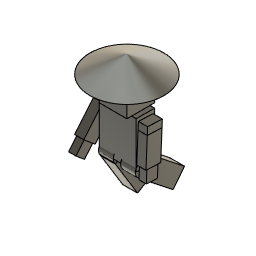
Body v3 (Autodesk Fusion 360 design; units mm, degrees)
Autodesk Fusion 360 part; units mm, degrees
sketch "Skizze2" plane through (0, 0, 0) normal (0, 0, 1) x (1, 0, 0)
  line L0 (-10, 5) -> (10, 5)
  line L1 (10, 5) -> (10, -5)
  line L2 (10, -5) -> (-10, -5)
  line L3 (-10, -5) -> (-10, 5)
  line L4 (-10, 0) -> (10, 0) construction
  line L5 (0, 5) -> (0, -5) construction
  dimension "d1" = 20
  dimension "d2" = 10
  constraint horizontal L0
  constraint vertical L1
  constraint horizontal L2
  constraint vertical L3
  constraint midpoint L3 L4.start
  constraint midpoint L1 L4.end
  constraint midpoint L0 L5.start
  constraint midpoint L2 L5.end
  constraint coincident origin L5
  constraint coincident origin L4
  measures "d1" distance of L0.start L0.end
  measures "d2" distance of L0 L2
extrude "Extrusion1" add sketch "Skizze2" along normal blind 25 makes body 1 in component "Body"
sketch "Skizze3" plane through (0, 0, 25) normal (0, 0, 1) x (-1, 0, 0)
  line L0 (10, 5) -> (-10, 5)
  line L1 (-10, 5) -> (-10, -5)
  line L2 (-10, -5) -> (10, -5)
  line L3 (10, -5) -> (10, 5)
  line L4 (7.5, -7.5) -> (-7.5, -7.5)
  line L5 (-7.5, -7.5) -> (-7.5, 7.5)
  line L6 (-7.5, 7.5) -> (7.5, 7.5)
  line L7 (7.5, 7.5) -> (7.5, -7.5)
  line L8 (0, -7.5) -> (0, 7.5) construction
  line L9 (7.5, 0) -> (-7.5, 0) construction
  dimension "d5" = 15
  dimension "d6" = 15
  constraint horizontal L4
  constraint vertical L5
  constraint horizontal L6
  constraint vertical L7
  constraint midpoint L4 L8.start
  constraint midpoint L6 L8.end
  constraint midpoint L7 L9.start
  constraint midpoint L5 L9.end
  constraint coincident origin L8
  constraint coincident origin L9
  measures "d5" distance of L4.start L4.end
  measures "d6" distance of L4.start L6.end
extrude "Extrusion1'" add sketch "Skizze3" along normal blind 15 separate body contours L0 L2 L5 L7 | L0 L5 L6 L7 | L2 L4 L5 L7 makes body 2 in component "Head"
sketch "Skizze4" plane through (0, 0, 0) normal (0, 0, -1) x (1, 0, 0)
  line L0 (10, 5) -> (-10, 5)
  line L1 (-10, 5) -> (-10, -5)
  line L2 (-10, -5) -> (10, -5)
  line L3 (10, -5) -> (10, 5)
  line L4 (-10, 0) -> (10, 0) construction
  line L5 (0, -5) -> (0, 5) construction
  line L6 (-10, 5) -> (-2, 5)
  line L7 (-2, 5) -> (-2, -5)
  line L8 (-2, -5) -> (-10, -5)
  line L9 (-10, -5) -> (-10, 5)
  line L10 (2, 5) -> (10, 5)
  line L11 (10, 5) -> (10, -5)
  line L12 (10, -5) -> (2, -5)
  line L13 (2, -5) -> (2, 5)
  line L14 (-10, 0) -> (-2, 0) construction
  line L15 (2, 0) -> (10, 0) construction
  dimension "d23" = 8
  dimension "d24" = 10
  dimension "d25" = 8
  dimension "d26" = 10
  constraint midpoint L1 L4.start
  constraint midpoint L3 L4.end
  constraint midpoint L2 L5.start
  constraint midpoint L0 L5.end
  constraint horizontal L6
  constraint vertical L7
  constraint horizontal L8
  constraint vertical L9
  constraint horizontal L10
  constraint vertical L11
  constraint horizontal L12
  constraint vertical L13
  constraint midpoint L9 L4.start
  constraint midpoint L7 L14.end
  constraint collinear L1 L9
  constraint collinear L4 L14
  constraint midpoint L13 L15.start
  constraint midpoint L11 L4.end
  constraint collinear L3 L11
  constraint collinear L4 L15
  measures "d23" distance of L0.end L6.end
  measures "d24" distance of L0.end L1.end
  measures "d25" distance of L10.start L0.start
  measures "d26" distance of L0.start L2.end
extrude "Extrusion1''" add sketch "Skizze4" along normal blind 28 separate body contours L0 L1 L2 L6 L7 L8 L9 makes body 3 in component "Leg left"
extrude "Extrusion1'''" add sketch "Skizze4" along normal blind 28 separate body contours L0 L2 L3 L10 L11 L12 L13 makes body 4 in component "Leg right"
sketch "Skizze5" plane through (10, 0, 0) normal (1, 0, 0) x (0, 1, 0)
  line L0 (-5, 0) -> (5, 0)
  line L1 (5, 0) -> (5, 25)
  line L2 (5, 25) -> (-5, 25)
  line L3 (-5, 25) -> (-5, 0)
  line L4 (-4, 23) -> (4, 23)
  line L5 (4, 23) -> (4, 3)
  line L6 (4, 3) -> (-4, 3)
  line L7 (-4, 3) -> (-4, 23)
  line L8 (0, 25) -> (0, 0) construction
  line L9 (-5, 12.5) -> (5, 12.5) construction
  line L10 (0, 23) -> (0, 3) construction
  line L11 (-4, 13) -> (4, 13) construction
  dimension "d31" = 8
  dimension "d32" = 20
  dimension "d35" = 2
  constraint horizontal L4
  constraint vertical L5
  constraint horizontal L6
  constraint vertical L7
  constraint midpoint L2 L8.start
  constraint coincident L8.end origin
  constraint midpoint L3 L9.start
  constraint midpoint L1 L9.end
  constraint midpoint L4 L10.start
  constraint midpoint L6 L10.end
  constraint midpoint L7 L11.start
  constraint midpoint L5 L11.end
  constraint collinear L8 L10
  measures "d31" distance of L4.start L4.end
  measures "d32" distance of L4.start L6.end
  measures "d35" distance of L2 L4
extrude "Extrusion1''''" add sketch "Skizze5" along normal blind 5 separate body contours L4 L5 L6 L7 makes body 5 in component "Arm right"
sketch "Skizze6" plane through (-10, 0, 0) normal (-1, 0, 0) x (0, -1, 0)
  line L0 (-5, 0) -> (5, 0)
  line L1 (5, 0) -> (5, 25)
  line L2 (5, 25) -> (-5, 25)
  line L3 (-5, 25) -> (-5, 0)
  line L4 (0, 25) -> (0, 0) construction
  line L5 (-5, 12.5) -> (5, 12.5) construction
  line L6 (-4, 23) -> (4, 23)
  line L7 (4, 23) -> (4, 3)
  line L8 (4, 3) -> (-4, 3)
  line L9 (-4, 3) -> (-4, 23)
  line L10 (0, 23) -> (0, 3) construction
  line L11 (-4, 13) -> (4, 13) construction
  dimension "d36" = 8
  dimension "d37" = 20
  dimension "d38" = 2
  constraint midpoint L2 L4.start
  constraint coincident L4.end origin
  constraint midpoint L3 L5.start
  constraint midpoint L1 L5.end
  constraint horizontal L6
  constraint vertical L7
  constraint horizontal L8
  constraint vertical L9
  constraint midpoint L6 L10.start
  constraint midpoint L8 L10.end
  constraint midpoint L9 L11.start
  constraint midpoint L7 L11.end
  constraint collinear L4 L10
  measures "d36" distance of L6.start L6.end
  measures "d37" distance of L6.end L7.end
  measures "d38" distance of L2 L6
extrude "Extrusion1'''''" add sketch "Skizze6" along normal blind 5 separate body contours L6 L7 L8 L9 makes body 6 in component "Arm left"
sketch "Skizze7" plane through (0, 0, 40) normal (0, 0, 1) x (-1, 0, 0)
  line L0 (7.5, 7.5) -> (-7.5, 7.5) construction
  line L1 (-7.5, 7.5) -> (-7.5, -7.5) construction
  line L2 (-7.5, -7.5) -> (7.5, -7.5) construction
  line L3 (7.5, -7.5) -> (7.5, 7.5) construction
  line L4 (7.5, 0) -> (-7.5, 0) construction
  line L5 (0, 7.5) -> (0, -7.5) construction
  constraint midpoint L3 L4.start
  constraint midpoint L1 L4.end
  constraint midpoint L0 L5.start
  constraint midpoint L2 L5.end
ref_plane "Arbeitsebene1" through (0, 0, 40) normal (0, -1, 0) x (1, 0, 0)
sketch "Skizze8" plane through (0, 0, 40) normal (0, -1, 0) x (1, 0, 0)
  line L0 (-7.5, 0) -> (7.5, 0)
  line L1 (0, -8.7843) -> (0, 12.5739) construction
  line L2 (0, 1) -> (-20, -1.6667)
  line L3 (-20, -1.6667) -> (0, 8)
  line L4 (0, 1) -> (0, 8)
  line L5 (-7.5, 0) -> (7.5, 0)
  point P0 (-7.5, 0)
  dimension "d42" = 7
  dimension "d43" = 8
  dimension "d44" = 20
  constraint perpendicular L0 L1
  constraint coincident origin L1
  constraint coincident L1 L2.start
  constraint coincident L1 L3.end
  constraint coincident L2 P0
  measures "d42" distance of L2.start L3.end
  measures "d43" distance of L3.end L5
  measures "d44" distance of L1 L2.end
revolve "Drehen1" add sketch "Skizze8" angle 360 about axis through (0, 0, 31.2157) along (0, 0, 1) separate body makes body 7 in component "Hut"
sketch "Skizze9" plane through (0, 0, 25) normal (0, 0, 1) x (-1, 0, 0)
  line L0 (10, 5) -> (-10, 5)
  line L1 (-10, 5) -> (-10, -5)
  line L2 (-10, -5) -> (10, -5)
  line L3 (10, -5) -> (10, 5)
  line L4 (3.5, -3.5) -> (-3.5, -3.5)
  line L5 (-3.5, -3.5) -> (-3.5, 3.5)
  line L6 (-3.5, 3.5) -> (3.5, 3.5)
  line L7 (3.5, 3.5) -> (3.5, -3.5)
  line L8 (10, 0) -> (-10, 0) construction
  line L9 (0, -5) -> (0, 5) construction
  line L10 (3.5, 0) -> (-3.5, 0) construction
  line L11 (0, -3.5) -> (0, 3.5) construction
  dimension "d48" = 7
  dimension "d49" = 7
  constraint horizontal L4
  constraint vertical L5
  constraint horizontal L6
  constraint vertical L7
  constraint midpoint L3 L8.start
  constraint midpoint L1 L8.end
  constraint midpoint L2 L9.start
  constraint midpoint L0 L9.end
  constraint midpoint L7 L10.start
  constraint midpoint L5 L10.end
  constraint midpoint L4 L11.start
  constraint midpoint L6 L11.end
  constraint collinear L8 L10
  constraint collinear L9 L11
  measures "d48" distance of L5.end L6.end
  measures "d49" distance of L4.start L6.end
extrude "Extrusion1''''''" add sketch "Skizze9" along normal blind 7.5 separate body contours L4 L5 L6 L7 makes body 8 in component "Hals"
combine "Kombinieren1" operation add target body 1 tool bodies 8 in component "Body"
sketch "Skizze10" plane through (0, 0, 3) normal (0, 0, -1) x (1, 0, 0)
  line L0 (-10, -4) -> (-10, 4)
  line L1 (-10, 4) -> (-15, 4)
  line L2 (-15, 4) -> (-15, -4)
  line L3 (-15, -4) -> (-10, -4)
  line L4 (-14.5, 3) -> (-10.5, 3)
  line L5 (-10.5, 3) -> (-10.5, -3)
  line L6 (-10.5, -3) -> (-14.5, -3)
  line L7 (-14.5, -3) -> (-14.5, 3)
  line L8 (-15, 0) -> (-10, 0) construction
  line L9 (-12.5, 4) -> (-12.5, -4) construction
  line L10 (-12.5, -3) -> (-12.5, 3) construction
  line L11 (-14.5, 0) -> (-10.5, 0) construction
  dimension "d55" = 6
  dimension "d56" = 4
  constraint horizontal L4
  constraint vertical L5
  constraint horizontal L6
  constraint vertical L7
  constraint midpoint L2 L8.start
  constraint midpoint L0 L8.end
  constraint midpoint L1 L9.start
  constraint midpoint L3 L9.end
  constraint midpoint L6 L10.start
  constraint midpoint L4 L10.end
  constraint midpoint L7 L11.start
  constraint midpoint L5 L11.end
  constraint collinear L9 L10
  constraint collinear L8 L11
  measures "d55" distance of L4.start L6.end
  measures "d56" distance of L4.start L4.end
extrude "Extrusion1'''''''" add sketch "Skizze10" along normal blind 7 separate body contours L4 L5 L6 L7 makes body 9 in component "Hand links"
sketch "Skizze11" plane through (0, 0, 3) normal (0, 0, -1) x (1, 0, 0)
  line L0 (10, 4) -> (10, -4)
  line L1 (10, -4) -> (15, -4)
  line L2 (15, -4) -> (15, 4)
  line L3 (15, 4) -> (10, 4)
  line L4 (10, 0) -> (15, 0) construction
  line L5 (12.5, 4) -> (12.5, -4) construction
  line L6 (10.5, 3) -> (14.5, 3)
  line L7 (14.5, 3) -> (14.5, -3)
  line L8 (14.5, -3) -> (10.5, -3)
  line L9 (10.5, -3) -> (10.5, 3)
  line L10 (10.5, 0) -> (14.5, 0) construction
  line L11 (12.5, 3) -> (12.5, -3) construction
  dimension "d59" = 4
  dimension "d60" = 6
  constraint midpoint L0 L4.start
  constraint midpoint L2 L4.end
  constraint midpoint L3 L5.start
  constraint midpoint L1 L5.end
  constraint horizontal L6
  constraint vertical L7
  constraint horizontal L8
  constraint vertical L9
  constraint midpoint L9 L10.start
  constraint midpoint L7 L10.end
  constraint midpoint L6 L11.start
  constraint midpoint L8 L11.end
  constraint collinear L4 L10
  constraint collinear L5 L11
  measures "d59" distance of L6.start L6.end
  measures "d60" distance of L6.end L7.end
extrude "Extrusion1''''''''" add sketch "Skizze11" along normal blind 7 separate body contours L6 L7 L8 L9 makes body 10 in component "Hand rechts"
combine "Kombinieren1'" operation add target body 6 tool bodies 9 in component "Arm left"
combine "Kombinieren1''" operation add target body 5 tool bodies 10 in component "Arm right"
sketch "Skizze12" plane through (-10, 14.0381, 4.6377) normal (1, 0, 0) x (0, 0.964453, 0.264253)
  line L0 (-17.8297, 3.1872) -> (-10.114, 1.0731) construction
  line L1 (-10.114, 1.0731) -> (-4.829, 20.3622) construction
  line L2 (-4.829, 20.3622) -> (-12.5446, 22.4762) construction
  line L3 (-12.5446, 22.4762) -> (-17.8297, 3.1872) construction
  line L4 (-12.5446, 22.4762) -> (-6.943, 12.6466) construction
  line L5 (-4.829, 20.3622) -> (-14.6586, 14.7606) construction
  line L6 (-4.829, 20.3622) -> (-12.5446, 22.4762) construction
  line L7 (-5.886, 16.5044) -> (-13.6016, 18.6184) construction
  point P0 (-9.7438, 17.5614)
  dimension "d73" = 45
  dimension "d74" = 45
  constraint coincident L2.end L3.start
  constraint coincident L1 L4.end
  constraint coincident L1.end L2.start
  constraint coincident L3 L5.end
  constraint midpoint L4 P0
  constraint coincident L1 L7.start
  constraint coincident L3 L7.end
  constraint perpendicular L3 L7
  constraint coincident P0 L7
  measures "d73" angle of L5 L6
  measures "d74" angle of L4 L6
sketch "Skizze13" plane through (10, 0, 0) normal (-1, 0, 0) x (0, -1, 0)
  line L0 (-4, 3) -> (4, 3) construction
  line L1 (4, 3) -> (4, 23) construction
  line L2 (4, 23) -> (-4, 23) construction
  line L3 (-4, 23) -> (-4, 3) construction
  line L4 (-4, 23) -> (4, 15) construction
  line L5 (4, 23) -> (-3.4948, 15.5052) construction
  point P0 (0, 19)
  dimension "d75" = 45
  dimension "d77" = 45
  constraint coincident L2.end L3.start
  constraint coincident L1 L4.end
  constraint coincident L1.end L2.start
  constraint midpoint L4 P0
  measures "d75" angle of L2 L4
  measures "d77" angle of L2 L5
sketch "Skizze14" plane through (10, 0, 0) normal (1, 0, 0) x (0, 1, 0)
  line L0 (-5, 0) -> (5, 0)
  line L1 (5, 0) -> (5, 25)
  line L2 (5, 25) -> (-5, 25)
  line L3 (-5, 25) -> (-5, 0)
  point P0 (0, 19)
sketch "Skizze15" plane through (-10, 0, 0) normal (-1, 0, 0) x (0, -1, 0)
  line L0 (-5, 0) -> (5, 0)
  line L1 (5, 0) -> (5, 25)
  line L2 (5, 25) -> (-5, 25)
  line L3 (-5, 25) -> (-5, 0)
  point P0 (0, 19)
ref_plane "Arbeitsebene2" through (-10, 0, 19) normal (0, 0, 1) x (0, -1, 0)
split "Teilen1" by plane through (-10, 0, 19) normal (0, 0, 1) bodies 6 makes body 11 at (-11.6667, 1.3333, 23) in component "Arm left"
split "Teilen1'" by plane through (-10, 0, 19) normal (0, 0, 1) bodies 5 makes body 12 at (11.6667, -1.3333, 23) in component "Arm right"
sketch "Skizze16" plane through (-10, 0, 0) normal (-1, 0, 0) x (0, -1, 0)
  line L0 (5, 0) -> (-5, 0) construction
  line L1 (-5, 0) -> (-5, -28) construction
  line L2 (-5, -28) -> (5, -28) construction
  line L3 (5, -28) -> (5, 0) construction
  line L4 (-5, 0) -> (5, -10) construction
  line L5 (5, 0) -> (-5, -10) construction
  line L6 (-5, -5) -> (5, -5) construction
  point P0 (0, -5)
  dimension "d87" = 45
  dimension "d88" = 45
  constraint coincident L0.end L1.start
  constraint coincident L3 L4.end
  constraint coincident L0.start L3.end
  constraint coincident L1 L5.end
  constraint midpoint L5 P0
  constraint coincident L1 L6.start
  constraint coincident L3 L6.end
  constraint perpendicular L3 L6
  constraint coincident P0 L6
  measures "d87" angle of L0 L5
  measures "d88" angle of L0 L4
ref_plane "Arbeitsebene3" through (-10, 0, -5) normal (0, 0, 1) x (0, -1, 0)
split "Teilen1''" by plane through (-10, 0, -5) normal (0, 0, 1) bodies 3 makes body 13 at (-7.3333, -1.6667, 0) in component "Leg left"
split "Teilen1'''" by plane through (-10, 0, -5) normal (0, 0, 1) bodies 4 makes body 14 at (4.6667, -1.6667, 0) in component "Leg right"
fillet "Abrundung1" radius 4 2 edges at (6, 5, 0) (6, -5, 0) on bodies 14 in component "Leg right"
fillet "Abrundung1'" radius 4 2 edges at (-6, -5, 0) (-6, 5, 0) on bodies 13 in component "Leg left"
component "Body" placed x (1, 0, 0) y (0, 1, 0) z (0, 0, 1) at (0, 0, 0)
component "Head" placed x (1, 0, 0) y (0, 1, 0) z (0, 0, 1) at (0, 0, 0)
component "Leg left" placed x (1, 0, 0) y (0, 1, 0) z (0, 0, 1) at (0, 0, 5)
component "Leg right" placed x (1, 0, 0) y (0, 1, 0) z (0, 0, 1) at (0, 0, 5)
component "Arm right" placed x (1, 0, 0) y (0, 1, 0) z (0, 0, 1) at (0, 0, 0)
component "Arm left" placed x (1, 0, 0) y (0, 1, 0) z (0, 0, 1) at (0, 0, 0)
component "Hut" placed x (1, 0, 0) y (0, 1, 0) z (0, 0, 1) at (0, 0, 0)
component "Hals" placed x (1, 0, 0) y (0, 1, 0) z (0, 0, 1) at (0, 0, 0)
component "Hand links" placed x (1, 0, 0) y (0, 1, 0) z (0, 0, 1) at (0, 0, 0)
component "Hand rechts" placed x (1, 0, 0) y (0, 1, 0) z (0, 0, 1) at (0, 0, 0)
equation "d1 = b_body"
equation "d2 = a_body"
equation "d3 = h_body"
equation "d5 = b_head"
equation "d6 = a_head"
equation "d7 = h_head"
equation "b_body = 20 mm"
equation "a_body = 10 mm"
equation "h_body = 25 mm"
equation "a_head = 15 mm"
equation "b_head = a_head"
equation "h_head = a_head"
equation "a_leg = 10 mm"
equation "b_leg = 8 mm"
equation "h_leg = 28 mm"
equation "a_arm = 8 mm"
equation "b_arm = 5 mm"
equation "h_arm = 20 mm"
equation "d23 = b_leg"
equation "d24 = a_leg"
equation "d25 = b_leg"
equation "d26 = a_leg"
equation "d27 = h_leg"
equation "d29 = h_leg"
equation "d31 = a_arm"
equation "d32 = h_arm"
equation "d33 = b_arm"
equation "d36 = a_arm"
equation "d37 = h_arm"
equation "d39 = b_arm"
equation "d42 = h_hat - 1 mm"
equation "d43 = h_hat"
equation "d44 = r_hat"
equation "a_neck = 7 mm"
equation "b_neck = a_neck"
equation "d48 = a_neck"
equation "d49 = b_neck"
equation "d50 = h_head / 2"
equation "a_hand = 4 mm"
equation "b_hand = 6 mm"
equation "h_hand = 7 mm"
equation "d55 = b_hand"
equation "d56 = a_hand"
equation "d57 = h_hand"
equation "d59 = a_hand"
equation "d60 = b_hand"
equation "d61 = h_hand"
equation "r_hat = 20 mm"
equation "h_hat = 8 mm"
equation "d91 = a_arm / 2"
equation "d93 = a_arm / 2"
